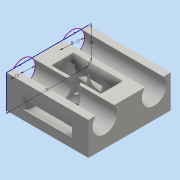
# Autodesk Inventor part: XCarriage
Saved by Autodesk Inventor 2016 (Build 200138000, 138)
## iProperties
Created: 2016-09-02
Part Number: XCarriage
Material: Generic
Document SubType Name: Modeling
Designer: Sam
Density: 1 g/cm^3
Appearance: Default
Author: Sam
Autodesk Inventor part; units mm, degrees
ref_plane "YZ Plane" through (0, 0, 0) normal (1, 0, 0) x (0, 1, 0)
ref_plane "XZ Plane" through (0, 0, 0) normal (0, 1, 0) x (-1, 0, 0)
ref_plane "XY Plane" through (0, 0, 0) normal (0, 0, 1) x (1, 0, 0)
sketch "Sketch2" plane through (0, 0, 0) normal (1, 0, 0) x (0, 1, 0)
  line L0 (0, 0) -> (4.4098, 0)
  line L1 (50, 0) -> (50, -20)
  line L2 (50, -20) -> (0, -20)
  line L3 (0, -20) -> (0, 0)
  circle A0 centre (10, -5) radius 7.5
  circle A1 centre (40, -5) radius 7.5
  arc A2 (25, 0) -> (50, -14) centre (41.5667, 0.262) ccw
  arc A3 (0, -14.4272) -> (25, 0) centre (8.4879, -0.2612) ccw
  arc A4 (0, -4.8915) -> (17.5, 0) centre (9.4336, -4.8915) ccw
  arc A5 (31, 0.262) -> (50, -4.8915) centre (40.0724, -3.8911) ccw
  line L4 (45.5902, 0) -> (50, 0)
  line L5 (34.4098, 0) -> (45.5902, 0)
  line L6 (30.8846, 0) -> (34.4098, 0)
  line L7 (25, 0) -> (30.8846, 0)
  line L8 (17.5, 0) -> (25, 0)
  line L9 (15.5902, 0) -> (17.5, 0)
  line L10 (4.4098, 0) -> (15.5902, 0)
  dimension "d22" = 50
  dimension "d23" = 20
  dimension "d24" = 15
  dimension "d25" = 15
  constraints: 22 end point, 13 point on circle, 9 parallel, 8 horizontal, 8 perpendicular, 6 centre point, 4 point on line, 2 tangent
  measures "d22" distance of L1.end L2.end
  measures "d23" distance of L1.start L1.end
  measures "d24" diameter of A0
  measures "d25" diameter of A1
extrude "Extrusion2" add sketch "Sketch2" along normal blind 10 contours L0 A0 L9 A4 L3 | A4 L8 A3 L3 | A3 A2 L1 L2 L3 | L7 A5 L1 A2 | L6 A1 L4 L1 A5
sketch "Sketch3" plane through (10, 0, 0) normal (1, 0, 0) x (0, 0, -1)
  line L0 (0, 0) -> (0, 4.4098)
  line L1 (0, 50) -> (20, 50)
  line L2 (20, 50) -> (20, 0)
  line L3 (20, 0) -> (0, 0)
  circle A0 centre (5, 10) radius 7.5
  circle A1 centre (5, 40) radius 7.5
  arc A2 (0, 25) -> (14, 50) centre (-0.262, 41.5667) ccw
  arc A3 (14.4272, 0) -> (0, 25) centre (0.2612, 8.4879) ccw
  arc A4 (4.8915, 0) -> (0, 17.5) centre (4.8915, 9.4336) ccw
  arc A5 (-0.262, 31) -> (4.8915, 50) centre (3.8911, 40.0724) ccw
  line L4 (0, 45.5902) -> (0, 50)
  line L5 (0, 34.4098) -> (0, 45.5902)
  line L6 (0, 30.8846) -> (0, 34.4098)
  line L7 (0, 25) -> (0, 30.8846)
  line L8 (0, 17.5) -> (0, 25)
  line L9 (0, 15.5902) -> (0, 17.5)
  line L10 (0, 4.4098) -> (0, 15.5902)
  dimension "d28" = 50
  dimension "d29" = 20
  dimension "d30" = 15
  dimension "d31" = 15
  constraints: 22 end point, 13 point on circle, 9 parallel, 8 perpendicular, 6 centre point, 4 point on line, 2 tangent
  measures "d28" distance of L1.end L2.end
  measures "d29" distance of L1.start L1.end
  measures "d30" diameter of A0
  measures "d31" diameter of A1
extrude "Extrusion3" add sketch "Sketch3" along normal blind 30 contours L0 A0 L9 A4 L3 | A3 A2 L1 L2 L3 | L6 A1 L4 L1 A5
sketch "Sketch4" plane through (40, 0, 0) normal (1, 0, 0) x (0, 0, -1)
  line L0 (0, 0) -> (0, 4.4098)
  line L1 (0, 50) -> (20, 50)
  line L2 (20, 50) -> (20, 0)
  line L3 (20, 0) -> (0, 0)
  circle A0 centre (5, 10) radius 7.5
  circle A1 centre (5, 40) radius 7.5
  arc A2 (0, 25) -> (14, 50) centre (-0.262, 41.5667) ccw
  arc A3 (14.4272, 0) -> (0, 25) centre (0.2612, 8.4879) ccw
  arc A4 (4.8915, 0) -> (0, 17.5) centre (4.8915, 9.4336) ccw
  arc A5 (-0.262, 31) -> (4.8915, 50) centre (3.8911, 40.0724) ccw
  line L4 (0, 45.5902) -> (0, 50)
  line L5 (0, 34.4098) -> (0, 45.5902)
  line L6 (0, 30.8846) -> (0, 34.4098)
  line L7 (0, 25) -> (0, 30.8846)
  line L8 (0, 17.5) -> (0, 25)
  line L9 (0, 15.5902) -> (0, 17.5)
  line L10 (0, 4.4098) -> (0, 15.5902)
  dimension "d34" = 50
  dimension "d35" = 20
  dimension "d36" = 15
  dimension "d37" = 15
  constraints: 22 end point, 13 point on circle, 9 parallel, 8 perpendicular, 6 centre point, 4 point on line, 2 tangent
  measures "d34" distance of L1.end L2.end
  measures "d35" distance of L1.start L1.end
  measures "d36" diameter of A0
  measures "d37" diameter of A1
extrude "Extrusion4" add sketch "Sketch4" along normal blind 10 contours L0 A0 L9 A4 L3 | A4 L8 A3 L3 | A3 A2 L1 L2 L3 | L7 A5 L1 A2 | L6 A1 L4 L1 A5
sketch "Sketch6" plane through (0, 15.5902, 0) normal (0, 0, 1) x (1, 0, 0)
  circle A0 centre (25, -1) radius 1.5
  line L0 (0, 0) -> (0, 50)
  circle A1 centre (29.5, 9) radius 1.5
  line L1 (40, 9) -> (10, 9)
  circle A2 centre (20.5, 9) radius 1.5
  point P0 (0, -15.5902)
  dimension "d47" = 3
  dimension "d48" = 25
  dimension "d49" = 3
  dimension "d50" = 4.5
  dimension "d51" = 10
  dimension "d52" = 3
  dimension "d53" = 4.5
  constraints: 4 end point, 3 centre point, 3 coincident, 1 point on line
  measures "d47" diameter of A0
  measures "d48" distance from line of L0 A0.centre
  measures "d49" diameter of A1
  measures "d50" horizontal distance of A0.centre A1.centre
  measures "d51" vertical distance of A0.centre A1.centre
  measures "d52" diameter of A2
  measures "d53" horizontal distance of A2.centre A0.centre
hole "Hole3" at (20.5, 24.5902, 0) at (29.5, 24.5902, 0) at (25, 14.5902, 0) direction (0, 0, -1) diameter 3.2 end through all counterbore diameter 8 counterbore depth 15
body "Solid2"
